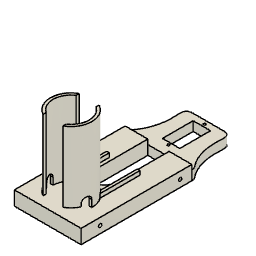
réservoir 1 euro (2) (Autodesk Fusion 360 design; units mm, degrees)
Autodesk Fusion 360 part; units mm, degrees
sketch "Base" plane through (0, 0, 0) normal (0, 1, 0) x (1, 0, 0)
  line L0 (-27.376, 9.2917) -> (22.624, 9.2917)
  line L1 (22.624, 9.2917) -> (22.624, -73.7083)
  line L2 (22.624, -73.7083) -> (-27.376, -73.7083)
  line L3 (-27.376, -73.7083) -> (-27.376, 9.2917)
  circle A0 centre (-2.376, -31.2083) radius 8
  line L4 (-10.376, 9.2917) -> (-10.376, -39.4326)
  line L5 (5.624, 9.2917) -> (5.624, -39.4326)
  dimension "d1_2" = 50
  dimension "d2_2" = 83
  dimension "d3_2" = 16
  dimension "d4_2" = 25
  dimension "d5_2" = 40.5
  constraint horizontal L0
  constraint vertical L1
  constraint horizontal L2
  constraint vertical L3
  constraint coincident L0 L4.start
  constraint perpendicular L0 L4
  constraint coincident L0 L5.start
  constraint perpendicular L0 L5
  constraint tangent A0 L4
  constraint tangent A0 L5
  measures "d1_2" distance of L0.start L0.end
  measures "d2_2" distance of L0.start L2.end
  measures "d3_2" diameter of A0
  measures "d4_2" distance of L1 A0.centre
  measures "d5_2" distance of L0 A0.centre
extrude "Extrude Base" add sketch "Base" along normal blind 10.6 contours L0 L1 L2 L3 A0 L4 L5
sketch "trous de centrage" plane through (0, 0, 0) normal (0, -1, 0) x (1, 0, 0)
  line L0 (5.624, -9.2917) -> (22.624, -9.2917)
  line L1 (22.624, -9.2917) -> (22.624, 73.7083)
  line L2 (22.624, 73.7083) -> (-27.376, 73.7083)
  line L3 (-27.376, 73.7083) -> (-27.376, -9.2917)
  line L4 (-27.376, -9.2917) -> (-10.376, -9.2917)
  line L5 (-10.376, -9.2917) -> (-10.376, 31.2083)
  arc A0 (5.624, 31.2083) -> (-10.376, 31.2083) centre (-2.376, 31.2083) ccw
  line L6 (5.624, 31.2083) -> (5.624, -9.2917)
  line L7 (-2.376, 73.7083) -> (-2.376, 54.2083) construction
  line L8 (1.124, 65.9583) -> (-5.876, 65.9583)
  line L9 (-5.876, 65.9583) -> (-5.876, 61.9583)
  line L10 (-5.876, 61.9583) -> (1.124, 61.9583)
  line L11 (1.124, 61.9583) -> (1.124, 65.9583)
  line L12 (1.124, 65.9583) -> (-5.876, 61.9583) construction
  line L13 (-5.876, 65.9583) -> (1.124, 61.9583) construction
  line L14 (-29.4384, 0.7083) -> (-4.6267, 0.7083) construction
  line L15 (-23.376, 9.0014) -> (-23.376, -13.8844) construction
  line L16 (-20.876, 4.2083) -> (-25.876, 4.2083)
  line L17 (-25.876, 4.2083) -> (-25.876, -2.7917)
  line L18 (-25.876, -2.7917) -> (-20.876, -2.7917)
  line L19 (-20.876, -2.7917) -> (-20.876, 4.2083)
  line L20 (-20.876, 4.2083) -> (-25.876, -2.7917) construction
  line L21 (-25.876, 4.2083) -> (-20.876, -2.7917) construction
  line L22 (21.124, -2.7917) -> (16.124, -2.7917)
  line L23 (16.124, -2.7917) -> (16.124, 4.2083)
  line L24 (16.124, 4.2083) -> (21.124, 4.2083)
  line L25 (21.124, 4.2083) -> (21.124, -2.7917)
  point P0 (-2.376, 63.9583)
  point P1 (-23.376, 0.7083)
  dimension "d27_2" = 7
  dimension "d28_2" = 4
  dimension "d29_2" = 10
  dimension "d30_2" = 4
  dimension "d31_2" = 7
  dimension "d32_2" = 5
  dimension "d122_2" = 9.75
  constraint midpoint L2 L7.start
  constraint perpendicular L8 L9
  constraint parallel L8 L10
  constraint parallel L9 L11
  constraint horizontal L8
  constraint coincident L12 P0
  constraint coincident L13 P0
  constraint midpoint L7 P0
  constraint perpendicular L5 L14
  constraint perpendicular L4 L15
  constraint perpendicular L16 L17
  constraint parallel L16 L18
  constraint parallel L17 L19
  constraint horizontal L16
  constraint coincident L20 P1
  constraint coincident L21 P1
  constraint coincident L15 P1
  constraint coincident L14 P1
  constraint symmetric L7 L16.start L23.end
  constraint symmetric L7 L16.end L24.end
  constraint symmetric L7 L17.end L22.start
  constraint symmetric L7 L18.end L22.end
  constraint vertical L7
  measures "d27_2" distance of L9.end L10.end
  measures "d28_2" distance of L8.end L9.end
  measures "d29_2" distance of L4 L14
  measures "d30_2" distance of L3 L15
  measures "d31_2" distance of L16.end L17.end
  measures "d32_2" distance of L17.end L18.end
  measures "d122_2" distance of L2 P0
extrude "Extrude trous de centrage" cut sketch "trous de centrage" against normal blind 3 contours L8 L9 L10 L11 | L16 L17 L18 L19 | L22 L23 L24 L25
chamfer "Chamfer trous de centrage" distance 2 angle 45 6 edges at (-5.876, 3, 63.9583) (1.124, 3, 63.9583) (21.124, 3, 0.7083) (16.124, 3, 0.7083) (-25.876, 3, 0.7083) (-20.876, 3, 0.7083)
sketch "Sketch1" plane through (0, 10.6, 0) normal (0, 1, 0) x (-1, 0, 0)
  line L0 (-22.624, -9.2917) -> (-5.624, -9.2917)
  line L1 (-5.624, -9.2917) -> (-5.624, 31.2083)
  arc A0 (10.376, 31.2083) -> (-5.624, 31.2083) centre (2.376, 31.2083) ccw
  line L2 (10.376, 31.2083) -> (10.376, -9.2917)
  line L3 (10.376, -9.2917) -> (27.376, -9.2917)
  line L4 (27.376, -9.2917) -> (27.376, 73.7083)
  line L5 (27.376, 73.7083) -> (-22.624, 73.7083)
  line L6 (-22.624, 73.7083) -> (-22.624, -9.2917)
  circle A1 centre (2.376, 56.2083) radius 13.5
  circle A2 centre (2.376, 56.2083) radius 15.5
  dimension "d20_2" = 27
  dimension "d21_2" = 31
  dimension "d22_2" = 17.5
  dimension "d23_2" = 25
  constraint concentric A1 A2
  measures "d20_2" diameter of A1
  measures "d21_2" diameter of A2
  measures "d22_2" distance of L5 A1.centre
  measures "d23_2" distance of L4 A1.centre
extrude "Extrude réservoir à pièces" add sketch "Sketch1" along normal blind 55.8 contours A2
sketch "Support servo" plane through (0, 0, 0) normal (0, -1, 0) x (1, 0, 0)
  line L0 (-5.876, 65.9583) -> (1.124, 65.9583)
  line L1 (1.124, 65.9583) -> (1.124, 61.9583)
  line L2 (1.124, 61.9583) -> (-5.876, 61.9583)
  line L3 (-5.876, 61.9583) -> (-5.876, 65.9583)
  line L4 (-25.876, 4.2083) -> (-20.876, 4.2083)
  line L5 (-20.876, 4.2083) -> (-20.876, -2.7917)
  line L6 (-20.876, -2.7917) -> (-25.876, -2.7917)
  line L7 (-25.876, -2.7917) -> (-25.876, 4.2083)
  line L8 (16.124, -2.7917) -> (16.124, 4.2083)
  line L9 (16.124, 4.2083) -> (21.124, 4.2083)
  line L10 (21.124, 4.2083) -> (21.124, -2.7917)
  line L11 (21.124, -2.7917) -> (16.124, -2.7917)
  line L12 (5.624, -9.2917) -> (22.624, -9.2917)
  line L13 (22.624, -9.2917) -> (22.624, 73.7083)
  line L14 (22.624, 73.7083) -> (-27.376, 73.7083)
  line L15 (-27.376, 73.7083) -> (-27.376, -9.2917)
  line L16 (-27.376, -9.2917) -> (-10.376, -9.2917)
  line L17 (-10.376, -9.2917) -> (-10.376, 31.2083)
  arc A0 (5.624, 31.2083) -> (-10.376, 31.2083) centre (-2.376, 31.2083) ccw
  line L18 (5.624, 31.2083) -> (5.624, -9.2917)
  line L19 (-8.376, -19.2917) -> (3.624, -19.2917) construction
  line L20 (3.624, -19.2917) -> (3.624, -41.2917) construction
  line L21 (3.624, -41.2917) -> (-8.376, -41.2917) construction
  line L22 (-8.376, -41.2917) -> (-8.376, -19.2917) construction
  line L23 (-8.876, -41.7917) -> (-8.876, -18.7917)
  line L24 (-8.876, -18.7917) -> (4.124, -18.7917)
  line L25 (4.124, -18.7917) -> (4.124, -41.7917)
  line L26 (4.124, -41.7917) -> (-8.876, -41.7917)
  line L27 (8.924, -46.5917) -> (-13.676, -46.5917)
  line L28 (-13.676, -46.5917) -> (-13.676, -13.9917)
  line L29 (-13.676, -13.9917) -> (8.924, -13.9917)
  line L30 (8.924, -13.9917) -> (8.924, -46.5917)
  line L31 (-2.376, -13.9917) -> (-2.376, -46.5917) construction
  circle A1 centre (-2.376, -43.7917) radius 0.9
  circle A2 centre (-2.376, -16.7917) radius 0.9
  line L32 (-13.676, -13.9917) -> (8.924, -13.9917)
  line L33 (8.924, -13.9917) -> (8.924, -9.2917)
  line L34 (8.924, -9.2917) -> (-13.676, -9.2917)
  line L35 (-13.676, -9.2917) -> (-13.676, -13.9917)
  line L36 (-2.376, 73.7083) -> (-2.376, -79.3696) construction
  spline S0 degree 5 poles (-13.676, -46.5917) (-14.6813, -46.5917) (-16.4026, -46.4093) (-18.1162, -45.5886) (-18.9006, -43.402) (-18.581, -38.9625) (-18.349, -33.0695) (-19.212, -26.3605) (-21.5908, -19.7176) (-24.1404, -15.1894) (-26.0746, -12.8238) (-26.9782, -11.7039) (-27.3035, -10.6666) (-27.376, -9.7821) (-27.376, -9.2917) knots 0 0 0 0 0 0 0.1 0.2 0.3 0.4 0.5 0.6 0.7 0.8 0.9 1 1 1 1 1 1
  line L37 (-10.2357, -46.5917) -> (-17.1162, -46.5917)
  line L38 (-18.5532, -28.3853) -> (-23.2263, -15.8038)
  line L39 (-27.376, -12.2236) -> (-27.376, -6.3598)
  spline S1 degree 5 poles (8.924, -46.5917) (9.9294, -46.5917) (11.6507, -46.4093) (13.3643, -45.5886) (14.1487, -43.402) (13.8291, -38.9625) (13.5971, -33.0695) (14.4601, -26.3605) (16.8389, -19.7176) (19.3885, -15.1894) (21.3227, -12.8238) (22.2262, -11.7039) (22.5516, -10.6666) (22.624, -9.7821) (22.624, -9.2917) knots 0 0 0 0 0 0 0.1 0.2 0.3 0.4 0.5 0.6 0.7 0.8 0.9 1 1 1 1 1 1
  line L40 (5.4838, -46.5917) -> (12.3643, -46.5917)
  line L41 (13.8013, -28.3853) -> (18.4744, -15.8038)
  line L42 (22.624, -12.2236) -> (22.624, -6.3598)
  point P0 (-20.8898, -22.0946)
  point P1 (16.1379, -22.0946)
  dimension "d37_2" = 12
  dimension "d38_2" = 22
  dimension "d39_2" = -0.5
  dimension "d40_2" = -5.3
  dimension "d41_2" = 1.8
  dimension "d42_2" = 1.8
  dimension "d43_2" = 2.5
  dimension "d44_2" = 2.5
  dimension "d45_2" = 4.7
  constraint horizontal L19
  constraint vertical L20
  constraint horizontal L21
  constraint vertical L22
  constraint midpoint L29 L31.start
  constraint midpoint L27 L31.end
  constraint coincident L31 A1.centre
  constraint coincident L31 A2.centre
  constraint horizontal L32
  constraint vertical L33
  constraint horizontal L34
  constraint vertical L35
  constraint collinear L30 L33
  constraint midpoint L14 L36.start
  constraint perpendicular L26 L36
  constraint collinear L31 L36
  constraint collinear L16 L34
  constraint symmetric L36 L27.end L27.start
  constraint symmetric L36 P0 P1
  constraint symmetric L36 L15.end L12.end
  constraint symmetric L36 L37.end L40.end
  constraint symmetric L36 L38.start L41.start
  constraint symmetric L36 L37.start L40.start
  constraint symmetric L36 L38.end L41.end
  constraint symmetric L36 L39.end L42.end
  constraint symmetric L36 L39.start L42.start
  measures "d37_2" distance of L19.start L19.end
  measures "d38_2" distance of L19.start L21.end
  measures "d41_2" diameter of A1
  measures "d42_2" diameter of A2
  measures "d43_2" distance of L19 A2.centre
  measures "d44_2" distance of L21 A1.centre
  measures "d45_2" distance of L28.end L34.end
extrude "Extrude3" add sketch "Support servo" against normal blind 7 contours L12 L16 L29 L32 L33 L34 L35 | L12 L30 L33 S1 | L27 L28 L29 L30 L32 L37 L40 | L16 L28 L35 S0
sketch "Sketch3" plane through (0, 66.4, 0) normal (0, 1, 0) x (-1, 0, 0)
  circle A0 centre (2.376, 56.2083) radius 13.5
  circle A1 centre (2.376, 56.2083) radius 15.5
  line L0 (2.376, 56.2083) -> (2.376, 87.487) construction
  line L1 (-5.124, 81.2083) -> (9.876, 81.2083)
  line L2 (9.876, 81.2083) -> (9.876, 31.2083)
  line L3 (9.876, 31.2083) -> (-5.124, 31.2083)
  line L4 (-5.124, 31.2083) -> (-5.124, 81.2083)
  line L5 (-5.124, 81.2083) -> (9.876, 31.2083) construction
  line L6 (9.876, 81.2083) -> (-5.124, 31.2083) construction
  point P0 (2.376, 56.2083)
  dimension "d48_2" = 50
  dimension "d49_2" = 15
  constraint coincident P0 A0.centre
  constraint vertical L0
  constraint perpendicular L1 L2
  constraint parallel L1 L3
  constraint parallel L2 L4
  constraint horizontal L1
  constraint coincident L5 P0
  constraint coincident L6 P0
  measures "d48_2" distance of L1.end L2.end
  measures "d49_2" distance of L2.end L3.end
extrude "Extrude4" cut sketch "Sketch3" against normal blind 55.8 contours A0 A1 L2 L4 | A0 A1 L2 L4
sketch "Passage du poussoir" plane through (0, 10.6, 0) normal (0, 1, 0) x (-1, 0, 0)
  arc A0 (-5.124, 69.7729) -> (-5.124, 42.6436) centre (2.376, 56.2083) ccw
  line L0 (-5.124, 69.7729) -> (-5.124, 67.4332)
  arc A1 (-5.124, 67.4332) -> (-5.124, 44.9833) centre (2.376, 56.2083) ccw
  line L1 (-5.124, 44.9833) -> (-5.124, 42.6436)
  line L2 (-22.624, -9.2917) -> (-5.624, -9.2917)
  line L3 (-5.624, -9.2917) -> (-5.624, 31.2083)
  arc A2 (10.376, 31.2083) -> (-5.624, 31.2083) centre (2.376, 31.2083) ccw
  line L4 (10.376, 31.2083) -> (10.376, -9.2917)
  line L5 (10.376, -9.2917) -> (27.376, -9.2917)
  line L6 (27.376, -9.2917) -> (27.376, 73.7083)
  line L7 (27.376, 73.7083) -> (-22.624, 73.7083)
  line L8 (-22.624, 73.7083) -> (-22.624, -9.2917)
  line L9 (9.876, 42.6436) -> (9.876, 44.9833)
  arc A3 (9.876, 44.9833) -> (9.876, 67.4332) centre (2.376, 56.2083) ccw
  line L10 (9.876, 67.4332) -> (9.876, 69.7729)
  arc A4 (9.876, 42.6436) -> (9.876, 69.7729) centre (2.376, 56.2083) ccw
  line L11 (2.376, 56.2083) -> (2.376, 73.7083) construction
  line L12 (-8.124, 41.2083) -> (12.876, 41.2083)
  line L13 (12.876, 41.2083) -> (12.876, 71.2083)
  line L14 (12.876, 71.2083) -> (-8.124, 71.2083)
  line L15 (-8.124, 71.2083) -> (-8.124, 41.2083)
  line L16 (-8.124, 41.2083) -> (12.876, 71.2083) construction
  line L17 (12.876, 41.2083) -> (-8.124, 71.2083) construction
  line L18 (27.376, 73.7083) -> (-22.624, 73.7083)
  line L19 (-22.624, 73.7083) -> (-22.624, 56.2083)
  line L20 (-22.624, 56.2083) -> (27.376, 56.2083)
  line L21 (27.376, 56.2083) -> (27.376, 73.7083)
  point P0 (2.376, 56.2083)
  dimension "d52_2" = 30
  dimension "d53_2" = 21
  dimension "d56_2" = 50
  dimension "d57_2" = 17.5
  constraint coincident P0 A0.centre
  constraint midpoint L7 L11.end
  constraint perpendicular L12 L13
  constraint parallel L12 L14
  constraint parallel L13 L15
  constraint horizontal L12
  constraint coincident L16 P0
  constraint coincident L17 P0
  constraint horizontal L18
  constraint vertical L19
  constraint horizontal L20
  constraint vertical L21
  constraint coincident L6.end L7.start
  measures "d52_2" distance of L12.end L13.end
  measures "d53_2" distance of L13.end L14.end
  measures "d56_2" distance of L6.end L7.end
  measures "d57_2" distance of L6.end L20.end
extrude "Extrude Passage poussoir" cut sketch "Passage du poussoir" along normal blind 3 contours A0 L0 A1 L15 | A0 L0 A1 A3 L10 A4 L13 L14 L15 L20 | A0 A1 L1 L15 | A0 A1 L1 L9 A3 A4 L12 L13 L15 L20 | A3 L10 A4 L13 | L9 A3 A4 L13
sketch "Sketch10" plane through (0, 10.6, 0) normal (0, 1, 0) x (-1, 0, 0)
  arc A0 (-8.124, 67.61) -> (-8.124, 44.8065) centre (2.376, 56.2083) ccw
  line L0 (-8.124, 67.61) -> (-8.124, 64.6936)
  line L1 (12.876, 44.8065) -> (12.876, 47.723)
  arc A1 (12.876, 44.8065) -> (12.876, 67.61) centre (2.376, 56.2083) ccw
  line L2 (-22.624, -9.2917) -> (-5.624, -9.2917)
  line L3 (-5.624, -9.2917) -> (-5.624, 31.2083)
  arc A2 (10.376, 31.2083) -> (-5.624, 31.2083) centre (2.376, 31.2083) ccw
  line L4 (10.376, 31.2083) -> (10.376, -9.2917)
  line L5 (10.376, -9.2917) -> (27.376, -9.2917)
  line L6 (27.376, -9.2917) -> (27.376, 73.7083)
  line L7 (27.376, 73.7083) -> (-22.624, 73.7083)
  line L8 (-22.624, 73.7083) -> (-22.624, -9.2917)
  line L9 (17.876, 72.7047) -> (-13.124, 72.7047)
  line L10 (-13.124, 72.7047) -> (-13.124, 56.2083)
  line L11 (-13.124, 56.2083) -> (17.876, 56.2083)
  line L12 (17.876, 56.2083) -> (17.876, 72.7047)
  line L13 (17.876, 72.7047) -> (-13.124, 56.2083) construction
  line L14 (-13.124, 72.7047) -> (17.876, 56.2083) construction
  line L15 (23.9426, 56.2083) -> (-19.297, 56.2083) construction
  arc A3 (-8.124, 64.6936) -> (-8.124, 47.723) centre (2.376, 56.2083) ccw
  line L16 (-8.124, 47.723) -> (-8.124, 44.8065)
  arc A4 (12.876, 47.723) -> (12.876, 64.6936) centre (2.376, 56.2083) ccw
  line L17 (12.876, 64.6936) -> (12.876, 67.61)
  point P0 (-13.124, 56.2083)
  dimension "d108_2" = 31
  constraint perpendicular L9 L10
  constraint parallel L9 L11
  constraint parallel L10 L12
  constraint horizontal L9
  constraint horizontal L15
  constraint coincident A0.centre L15
  constraint midpoint A0 P0
  constraint coincident P0 L10.end
  measures "d108_2" distance of P0 L11.end
extrude "Extrude passage pièce" cut sketch "Sketch10" along normal blind 3 contours A0 L0 L11 A3 | A1 L11 A4 L17
sketch "Guide poussoir" plane through (0, 10.6, 0) normal (0, 1, 0) x (-1, 0, 0)
  line L0 (-22.624, -9.2917) -> (-5.624, -9.2917)
  line L1 (-5.624, -9.2917) -> (-5.624, 31.2083)
  arc A0 (10.376, 31.2083) -> (-5.624, 31.2083) centre (2.376, 31.2083) ccw
  line L2 (10.376, 31.2083) -> (10.376, -9.2917)
  line L3 (10.376, -9.2917) -> (27.376, -9.2917)
  line L4 (27.376, -9.2917) -> (27.376, 73.7083)
  line L5 (27.376, 73.7083) -> (-22.624, 73.7083)
  line L6 (-22.624, 73.7083) -> (-22.624, -9.2917)
  line L7 (14.876, 17.0431) -> (-10.124, 17.0431)
  line L8 (-10.124, 17.0431) -> (-10.124, 47.0431)
  line L9 (-10.124, 47.0431) -> (14.876, 47.0431)
  line L10 (14.876, 47.0431) -> (14.876, 17.0431)
  line L11 (12.876, 17.0431) -> (-8.124, 17.0431)
  line L12 (-8.124, 17.0431) -> (-8.124, 47.0431)
  line L13 (-8.124, 47.0431) -> (12.876, 47.0431)
  line L14 (12.876, 47.0431) -> (12.876, 17.0431)
  arc A1 (-13.124, 56.2083) -> (-8.124, 44.8065) centre (2.376, 56.2083) ccw
  line L15 (-13.124, 56.2083) -> (-11.124, 56.2083)
  line L16 (-8.124, 47.723) -> (-8.124, 44.8065)
  line L17 (12.876, 44.8065) -> (12.876, 47.723)
  line L18 (15.876, 56.2083) -> (17.876, 56.2083)
  arc A2 (12.876, 44.8065) -> (17.876, 56.2083) centre (2.376, 56.2083) ccw
  arc A3 (-11.124, 56.2083) -> (-8.124, 47.723) centre (2.376, 56.2083) ccw
  arc A4 (12.876, 47.723) -> (15.876, 56.2083) centre (2.376, 56.2083) ccw
  point P0 (-10.124, 47.0431)
  dimension "d111_2" = 25
  dimension "d112_2" = 30
  dimension "d113_2" = 21
  dimension "d114_2" = 30
  dimension "d115_2" = 2
  dimension "d149_2" = 12.5
  constraint horizontal L7
  constraint vertical L8
  constraint horizontal L9
  constraint vertical L10
  constraint horizontal L11
  constraint vertical L12
  constraint horizontal L13
  constraint vertical L14
  constraint collinear L9 L13
  constraint coincident L8 P0
  constraint coincident P0 L8.end
  constraint coincident L9.end A2
  measures "d111_2" distance of L7.start L7.end
  measures "d112_2" distance of L7.start L9.end
  measures "d113_2" distance of L11.start L11.end
  measures "d114_2" distance of L11.start L13.end
  measures "d115_2" distance of L10 L14
  measures "d149_2" distance of L4 L7.start
extrude "Extrude7" add sketch "Guide poussoir" along normal blind 3 contours L7 L8 L12 A1 | L7 L10 L14 A2 | L9 L12 A1 L16 | L9 L14 L17 A2
sketch "Trou de vis et passage tournevis" plane through (22.624, 0, 0) normal (1, 0, 0) x (0, 0, -1)
  line L0 (-73.7083, 0) -> (9.2917, 0)
  line L1 (9.2917, 0) -> (9.2917, 7)
  line L2 (9.2917, 7) -> (9.2917, 10.6)
  line L3 (9.2917, 10.6) -> (-73.7083, 10.6)
  line L4 (-73.7083, 10.6) -> (-73.7083, 0)
  line L5 (-76.6398, 15.9) -> (-29.5985, 15.9) construction
  circle A0 centre (-59.4583, 15.9) radius 3.25
  circle A1 centre (-59.4583, 5.3) radius 1.25
  line L6 (-59.4583, 25.6832) -> (-59.4583, -3.9867) construction
  line L7 (-4.2083, 3) -> (2.7917, 3) construction
  line L8 (-4.2083, 3) -> (2.7917, 3) construction
  circle A2 centre (0.5417, 5.3) radius 1.25
  line L9 (0.5417, 2.7793) -> (0.5417, 9.3839) construction
  line L10 (-73.7083, 5.3) -> (9.2917, 5.3) construction
  line L11 (46.5917, 0) -> (46.5917, 7)
  line L12 (-67.4332, 13.6) -> (-67.4332, 66.4)
  line L13 (-62.7083, 15.9) -> (-62.7083, 10.6)
  line L14 (-56.2083, 10.6) -> (-62.7083, 10.6)
  line L15 (-56.2083, 15.9) -> (-56.2083, 10.6)
  line L16 (-56.2083, 13.6) -> (-56.2083, 10.6)
  point P0 (-0.7083, 3)
  dimension "d71_2" = 5.3
  dimension "d72_2" = 6.5
  dimension "d76_2" = 2.5
  dimension "d77_2" = 2.5
  dimension "d101_2" = 60
  dimension "d105_2" = 6.8
  dimension "d117_2" = 45.8
  constraint horizontal L5
  constraint coincident L5 A0.centre
  constraint perpendicular L5 L6
  constraint coincident A0.centre L6
  constraint coincident A1.centre L6
  constraint horizontal L7
  constraint equal L7 L8
  constraint collinear L7 L8
  constraint coincident L7.start L8.start
  constraint midpoint L8 P0
  constraint perpendicular L8 L9
  constraint coincident A2.centre L9
  constraint midpoint L4 L10.start
  constraint coincident L1 L10.end
  constraint perpendicular L1 L10
  constraint coincident A1.centre L10
  constraint coincident A2.centre L10
  constraint coincident L5 L13.start
  constraint coincident A0 L13.start
  constraint tangent A0 L13
  constraint collinear L3 L14
  constraint coincident L5 L15.start
  constraint coincident L3 L14.start
  constraint perpendicular L3 L15
  constraint tangent A0 L15
  constraint coincident L14.start L15.end
  constraint collinear L15 L16
  measures "d71_2" distance of L3 L5
  measures "d72_2" diameter of A0
  measures "d76_2" diameter of A1
  measures "d77_2" diameter of A2
  measures "d101_2" distance of A1.centre L9
extrude "Extrude trou de vis" cut sketch "Trou de vis et passage tournevis" against normal blind 16 contours A1 | A2
extrude "Extrude passage tournevis" cut sketch "Trou de vis et passage tournevis" against normal blind 48 contours L3 A0 L13 L14 L15 L16 | A0
equation "d20_2 = Piece2euros"
equation "d72_2 = DiamTournevis"
equation "d76_2 = perçageO3"
equation "d77_2 = perçageO3"
equation "d122_2 = 10 mm - 0.25 mm"
equation "d149_2 = ( ( 50 - 25 ) / 2 ) * 1 mm"
equation "Piece2euros = 27 mm"
equation "DiamTournevis = 6.5 mm"
equation "perçageO3 = 2.5 mm"
